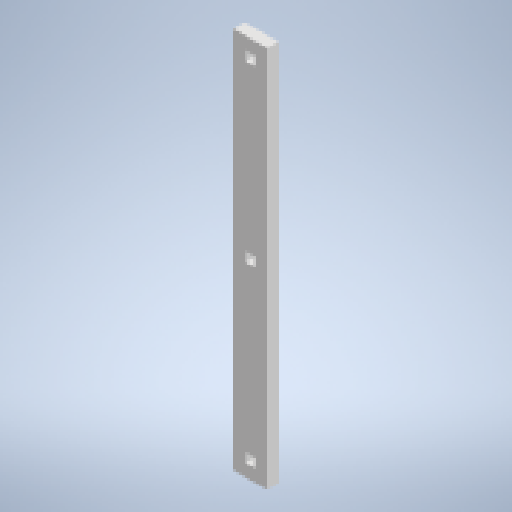
# Autodesk Inventor part: BareCalibrationClipFeet
Saved by Autodesk Inventor 2024 (Build 280153000, 153)
## iProperties
Created: 2024-03-12
Part Number: BareCalibrationClipFeet
Material: Generic
Document SubType Name: Modeling
Designer: jevan
Density: 1 g/cm^3
Appearance: Default
Author: jevan
Autodesk Inventor part; units mm, degrees
ref_plane "YZ Plane" through (0, 0, 0) normal (1, 0, 0) x (0, 1, 0)
ref_plane "XZ Plane" through (0, 0, 0) normal (0, 1, 0) x (-1, 0, 0)
ref_plane "XY Plane" through (0, 0, 0) normal (0, 0, 1) x (1, 0, 0)
sketch "Sketch1" plane through (0, 0, 0) normal (0, 0, 1) x (1, 0, 0)
  line L0 (2.05, 2.05) -> (-2.05, 2.05)
  line L1 (-2.05, 2.05) -> (-2.05, -2.05)
  line L2 (-2.05, -2.05) -> (2.05, -2.05)
  line L3 (2.05, -2.05) -> (2.05, 2.05)
  line L4 (7.5, -85) -> (-7.5, -85)
  line L5 (-7.5, -85) -> (-7.5, 85)
  line L6 (-7.5, 85) -> (7.5, 85)
  line L7 (7.5, 85) -> (7.5, -85)
  line L8 (25, 85) -> (-25, 85)
  line L9 (-25, 85) -> (-25, 75)
  line L10 (-25, 75) -> (25, 75)
  line L11 (25, 75) -> (25, 85)
  line L12 (7.5, 0) -> (-7.5, 0)
  line L13 (-7.5, -85) -> (7.5, -85)
  line L14 (25, -85) -> (-25, -85)
  line L15 (-25, -85) -> (-25, -75)
  line L16 (-25, -75) -> (25, -75)
  line L17 (25, -75) -> (25, -85)
  arc A0 (25, 75) -> (25, -75) centre (176.9643, 0) ccw
  arc A1 (-25, -75) -> (-25, 75) centre (-176.9643, 0) ccw
  point P0 (0, 0)
  point P1 (-7.5, -85)
  point P2 (7.5, 85)
  dimension "d0" = 4.1
  dimension "d1" = 4.1
  dimension "d2" = 2.05
  dimension "d3" = 2.05
  dimension "d4" = 170
  dimension "d5" = 15
  dimension "d6" = 7.5
  dimension "d7" = 85
  dimension "d18" = 50
  dimension "d19" = 25
  dimension "d20" = 10
  constraints: 36 end point, 6 parallel, 6 point on circle, 4 symmetric about line, 3 horizontal, 3 perpendicular, 2 centre point, 2 midpoint, 1 collinear
  measures "d0" distance of L2.end L1.end
  measures "d1" distance of L1.end L0.end
  measures "d2" distance from line of L3 point (0, 0)
  measures "d3" distance from line of L2 point (0, 0)
  measures "d4" distance of L4.end L5.end
  measures "d5" distance between parallel lines of L7 L5
  measures "d6" distance from line of L7 point (0, 0)
  measures "d7" distance from line of L4 point (0, 0)
  measures "d18" distance between parallel lines of L9 L11
  measures "d19" distance from line of point (0, 0) L9
  measures "d20" distance between parallel lines of L8 L10
extrude "Extrusion1" add sketch "Sketch1" along normal blind 5
extrude "Extrusion2" cut sketch "Sketch1" along normal blind 4.1 contours L3 L12 L1 L0 | L3 L2 L1 L12
pattern_linear "Rectangular Pattern1" count 3 spacing 77.3598 along (0, 1, 0) of "Extrusion2" first direction both ways yes
chamfer "Chamfer1" distance 0.5 angle 45 12 edges at (2.05, 77.3598, 0) (0, 79.4098, 0) (-2.05, 77.3598, 0) (0, 75.3098, 0) (0, -2.05, 0) (2.05, 0, 0) (0, 2.05, 0) (-2.05, 0, 0) (0, -79.4098, 0) (-2.05, -77.3598, 0) (0, -75.3098, 0) (2.05, -77.3598, 0)
equation "\"d1\" = d0"
equation "\"d2\" = 0.5 * d0"
equation "\"d3\" = 0.5 * d0"
equation "\"d6\" = 0.5 * d5"
equation "\"d7\" = 0.5 * d4"
equation "\"d19\" = 0.5 * d18"
body "Solid1"
